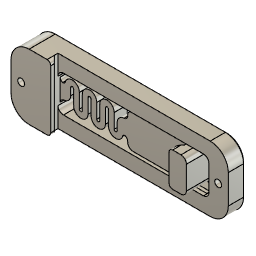
pcb_din_clip_x3 (Autodesk Fusion 360 design; units mm, degrees)
Autodesk Fusion 360 part; units mm, degrees
sketch "Sketch1" plane through (0, 0, 0) normal (0, 0, 1) x (1, 0, 0)
  line L0 (28.45, -9) -> (-28.45, -9)
  line L1 (-28.45, -9) -> (-28.45, 9)
  line L2 (-28.45, 9) -> (28.45, 9)
  line L3 (28.45, 9) -> (28.45, -9)
  line L4 (28.45, -9) -> (-28.45, 9) construction
  line L5 (-28.45, -9) -> (28.45, 9) construction
  dimension "d432" = 56.9
  dimension "d433" = 18
  constraint horizontal L0
  constraint perpendicular L0 L1
  constraint parallel L0 L2
  constraint parallel L1 L3
  constraint coincident L4 origin
  constraint coincident L5 origin
  measures "d432" distance of L1.end L2.end
  measures "d433" distance of L0.start L2.end
extrude "Extrude1" add sketch "Sketch1" along normal blind 7.6
sketch "Sketch2" plane through (0, 0, 7.6) normal (0, 0, 1) x (1, 0, 0)
  line L0 (28.45, 9) -> (-28.45, 9)
  line L1 (-28.45, 9) -> (-28.45, -9)
  line L2 (-28.45, -9) -> (28.45, -9)
  line L3 (28.45, -9) -> (28.45, 9)
  line L4 (-17.5, 9) -> (28.45, 9)
  line L5 (28.45, 9) -> (28.45, -9)
  line L6 (28.45, -9) -> (-17.5, -9)
  line L7 (-17.5, -9) -> (-17.5, 9)
  dimension "d436" = 10.95
  constraint horizontal L4
  constraint vertical L5
  constraint horizontal L6
  constraint vertical L7
  constraint coincident L2.end L3.start
  constraint coincident L0 L4.start
  measures "d436" distance of L1 L7
extrude "Extrude2" cut sketch "Sketch2" against normal blind 3 contours L0 L2 L3 L4 L5 L6 L7
sketch "Sketch3" plane through (0, -9, 0) normal (0, -1, 0) x (1, 0, 0)
  line L0 (28.45, 4.6) -> (-17.5, 4.6)
  line L1 (-17.5, 4.6) -> (-17.5, 7.6)
  line L2 (-17.5, 7.6) -> (-28.45, 7.6)
  line L3 (-28.45, 7.6) -> (-28.45, 0)
  line L4 (-28.45, 0) -> (28.45, 0)
  line L5 (28.45, 0) -> (28.45, 4.6)
  line L6 (-17.5, 6.6) -> (-18.5, 5.6)
  line L7 (-18.5, 5.6) -> (-18.5, 4.6)
  line L8 (-18.5, 4.6) -> (-17.5, 4.6)
  dimension "d439" = 1
  dimension "d440" = 1
  constraint coincident L1 L6.start
  constraint perpendicular L0 L7
  constraint coincident L0.end L1.start
  constraint perpendicular L1 L8
  constraint equal L7 L8
  measures "d439" distance of L7.end L0.end
  measures "d440" distance of L2 L6.start
extrude "Extrude3" cut sketch "Sketch3" against normal through all contours L1 L6 L7 L8
sketch "Sketch4" plane through (0, 0, 0) normal (0, 0, -1) x (-1, 0, 0)
  line L0 (28.45, 9) -> (-28.45, 9)
  line L1 (-28.45, 9) -> (-28.45, -9)
  line L2 (-28.45, -9) -> (28.45, -9)
  line L3 (28.45, -9) -> (28.45, 9)
  line L4 (-23.1, 5) -> (18.5, 5)
  line L5 (18.5, 5) -> (18.5, -5)
  line L6 (18.5, -5) -> (-23.1, -5)
  line L7 (-23.1, -5) -> (-23.1, 5)
  line L8 (-23.1, 5) -> (18.5, -5) construction
  line L9 (18.5, 5) -> (-23.1, -5) construction
  point P0 (-2.3, 0)
  dimension "d506" = 0.4
  constraint horizontal L4
  constraint perpendicular L4 L5
  constraint parallel L4 L6
  constraint parallel L5 L7
  constraint coincident L8 P0
  constraint coincident L9 P0
  constraint horizontal origin P0
  measures "d442" distance of L5.end L6.end
  measures "d443" distance of L1 L7
  measures "d453" distance of L4.start L6.end
extrude "Extrude4" cut sketch "Sketch4" against normal up to surface (4.6 mm away) contours L4 L5 L6 L7
ref_plane "WorkPlane1" through (21.5, 0, 3.8) normal (1, 0, 0) x (0, 1, 0)
sketch "Sketch5" plane through (21.5, 0, 2.1) normal (1, 0, 0) x (0, 0, -1)
  line L0 (0.4655, 6) -> (-0.4655, 6)
  line L1 (-0.4655, 6) -> (-0.4655, -6)
  line L2 (-0.4655, -6) -> (0.4655, -6)
  line L3 (0.4655, -6) -> (0.4655, 6)
  line L4 (0.4655, 6) -> (-0.4655, -6) construction
  line L5 (-0.4655, 6) -> (0.4655, -6) construction
  dimension "d447" = 0.931
  dimension "d448" = 12
  constraint horizontal L0
  constraint perpendicular L0 L1
  constraint parallel L0 L2
  constraint parallel L1 L3
  constraint coincident L4 origin
  constraint coincident L5 origin
  measures "d447" distance of L0.start L0.end
  measures "d448" distance of L0.start L2.end
extrude "Extrude5" cut sketch "Sketch5" against normal blind 15.5
chamfer "Chamfer1" distance 1 angle 45 4 edges at (13.75, 5, 2.5655) (13.75, 5, 1.6345) (13.75, -5, 2.5655) (13.75, -5, 1.6345)
sketch "Sketch6" plane through (0, 0, 0) normal (0, 0, -1) x (-1, 0, 0)
  line L0 (-23.1, -5) -> (-23.1, 5)
  line L1 (-23.1, 5) -> (18.5, 5)
  line L2 (18.5, 5) -> (18.5, -5)
  line L3 (18.5, -5) -> (-23.1, -5)
  line L4 (28.45, 9) -> (-28.45, 9)
  line L5 (-28.45, 9) -> (-28.45, -9)
  line L6 (-28.45, -9) -> (28.45, -9)
  line L7 (28.45, -9) -> (28.45, 9)
  line L8 (18.5, 5) -> (18.5, -5)
  line L9 (-23.1, 5) -> (18.5, 5)
  line L10 (18.5, -5) -> (-23.1, -5)
  line L11 (-23.1, -5) -> (-23.1, 5)
  line L12 (18.5, -2) -> (15.6, -2)
  line L13 (15.6, -2) -> (15.6, 2)
  line L14 (17.2, 2) -> (18.5, 2)
  line L15 (18.5, 2) -> (18.5, -2)
  line L16 (18.5, -2) -> (15.6, 2) construction
  line L17 (15.6, -2) -> (18.5, 2) construction
  line L18 (13.2, 2) -> (13.2, -2)
  line L19 (14.8, 2) -> (14.8, -2)
  arc A0 (10.8, -2) -> (14.8, -2) centre (12.8, -2) ccw
  arc A1 (17.2, 2) -> (13.2, 2) centre (15.2, 2) ccw
  line L20 (12.4, 2) -> (12.4, -2)
  line L21 (10.8, -2) -> (10.8, 2)
  arc A2 (12.4, -2) -> (13.2, -2) centre (12.8, -2) ccw
  arc A3 (12.4, 2) -> (8.4, 2) centre (10.4, 2) ccw
  line L22 (8.4, 2) -> (8.4, 2)
  arc A4 (15.6, 2) -> (14.8, 2) centre (15.2, 2) ccw
  arc A5 (10.8, 2) -> (10, 2) centre (10.4, 2) ccw
  line L23 (10, 2) -> (10, -2)
  line L24 (8.4, 2) -> (8.4, -2)
  arc A6 (6, -2) -> (10, -2) centre (8, -2) ccw
  line L25 (7.6, -2) -> (7.6, 2)
  line L26 (6, -2) -> (6, 2)
  arc A7 (7.6, -2) -> (8.4, -2) centre (8, -2) ccw
  line L27 (5.2, 2) -> (5.2, -2)
  line L28 (3.6, 2) -> (3.6, -2)
  line L29 (1.2, -2) -> (-0.1, -2)
  line L30 (-0.1, -2) -> (-0.1, 2)
  line L31 (-0.1, 2) -> (2.8, 2)
  line L32 (2.8, 2) -> (2.8, -2)
  line L33 (2.8, -2) -> (-0.1, 2) construction
  line L34 (-0.1, -2) -> (2.8, 2) construction
  arc A8 (1.2, -2) -> (5.2, -2) centre (3.2, -2) ccw
  arc A9 (7.6, 2) -> (3.6, 2) centre (5.6, 2) ccw
  arc A10 (6, 2) -> (5.2, 2) centre (5.6, 2) ccw
  arc A11 (2.8, -2) -> (3.6, -2) centre (3.2, -2) ccw
  arc A12 (10.8, 2.0006) -> (10, 1.9994) centre (10.4, 2) ccw
  arc A13 (10.8, 1.9994) -> (10.8, 2) centre (10.4, 2) ccw
  line L35 (-0.1, -4.7) -> (-19.9, -4.7)
  line L36 (-19.9, -4.7) -> (-19.9, 4.7)
  line L37 (-19.9, 4.7) -> (-0.1, 4.7)
  line L38 (-0.1, 4.7) -> (-0.1, -4.7)
  line L39 (-0.1, -4.7) -> (-19.9, 4.7) construction
  line L40 (-19.9, -4.7) -> (-0.1, 4.7) construction
  point P0 (17.05, 0)
  point P1 (1.35, 0)
  point P2 (-10, 0)
  dimension "d456" = 2.9
  dimension "d457" = 4
  dimension "d458" = 4
  dimension "d464" = 0.8
  dimension "d465" = 2.9
  dimension "d466" = 4
  dimension "d469" = 19.8
  dimension "d470" = 9.4
  constraint horizontal L12
  constraint perpendicular L12 L13
  constraint parallel L12 L14
  constraint parallel L13 L15
  constraint coincident L16 P0
  constraint coincident L17 P0
  constraint horizontal origin P0
  constraint coincident L8 L14.end
  constraint coincident L14 A1.centre
  constraint equal A0 A1
  constraint concentric A0 A2
  constraint coincident L12 A0.centre
  constraint tangent L18 A2
  constraint vertical L18
  constraint tangent L19 A0
  constraint vertical L19
  constraint concentric A3 A5
  constraint equal A1 A3
  constraint horizontal A1.centre A3.centre
  constraint tangent L20 A2
  constraint vertical L21
  constraint vertical L20
  constraint perpendicular L21 L22
  constraint horizontal A3.centre L21.end
  constraint horizontal L13.end L14.start
  constraint tangent L13 A4
  constraint horizontal L13.end A1.centre
  constraint tangent L19 A4
  constraint coincident A1.centre A4.centre
  constraint tangent L18 A1
  constraint coincident L21 A12.start
  constraint concentric A5 A12
  constraint concentric A6 A7
  constraint equal A0 A6
  constraint equal A2 A7
  constraint tangent L20 A3
  constraint tangent L21 A5
  constraint tangent A5 L23
  constraint vertical L24
  constraint horizontal A0.centre A6.centre
  constraint tangent L23 A6
  constraint vertical L23
  constraint concentric A9 A10
  constraint equal A3 A9
  constraint equal A5 A10
  constraint vertical L25
  constraint vertical L26
  constraint tangent A6 L26
  constraint tangent L25 A9
  constraint tangent L24 A7
  constraint tangent L25 A7
  constraint horizontal A3.centre A9.centre
  constraint vertical L27
  constraint vertical L28
  constraint tangent L27 A10
  constraint tangent L28 A9
  constraint horizontal L29
  constraint perpendicular L29 L30
  constraint parallel L29 L31
  constraint parallel L30 L32
  constraint coincident L33 P1
  constraint coincident L34 P1
  constraint horizontal origin P1
  constraint tangent L27 A8
  constraint equal A7 A11
  constraint coincident A8.centre A11.centre
  constraint tangent L28 A11
  constraint tangent L32 A11
  constraint horizontal L32.end L29.end
  constraint vertical L32.end L33.start
  constraint horizontal L29.start L32.end
  constraint coincident L23 A12.end
  constraint coincident L21 A13.start
  constraint concentric A12 A13
  constraint horizontal L35
  constraint perpendicular L35 L36
  constraint parallel L35 L37
  constraint parallel L36 L38
  constraint coincident L39 P2
  constraint coincident L40 P2
  constraint horizontal P1 P2
  constraint coincident L30.end L38
  measures "d456" distance of L12.start L12.end
  measures "d457" distance of L12.start L14.end
  measures "d458" diameter of A1
  measures "d464" diameter of A4
  measures "d465" distance of L32.end L29.end
  measures "d466" distance of L29.end L30.end
  measures "d469" distance of L36.end L37.end
  measures "d470" distance of L35.end L36.end
extrude "Extrude6" add sketch "Sketch6" against normal blind 4 contours L2 L8 L12 L13 L14 L15 L18 L19 A0 A1 L20 L21 A2 A3 A4 A5 L23 L24 A6 L25 L26 A7 L27 L28 L29 L30 L31 L32 A8 A9 A10 A11 A12 A13 L38 | L30 L35 L36 L37 L38
ref_plane "WorkPlane2" through (17.3, 0, 2) normal (1, 0, 0) x (0, 1, 0)
sketch "Sketch7" plane through (17.3, 0, 2) normal (1, 0, 0) x (0, 0, -1)
  line L0 (-0.4, -5.7) -> (0.2, -5.7)
  line L1 (0.2, -5.7) -> (0.2, 5.7)
  line L2 (0.2, 5.7) -> (-0.4, 5.7)
  line L3 (-0.4, 5.7) -> (-0.4, -5.7)
  line L4 (-0.4, -5.7) -> (0.2, 5.7) construction
  line L5 (0.2, -5.7) -> (-0.4, 5.7) construction
  line L6 (2, 4.7) -> (-2, 4.7)
  line L7 (2, -4.7) -> (-2, -4.7)
  line L8 (0.2, 5.7) -> (1.2, 4.7)
  line L9 (-0.4, 5.7) -> (-1.4, 4.7)
  line L10 (-1.4, 4.7) -> (-0.4, 4.7)
  line L11 (0.2, -5.7) -> (1.2, -4.7)
  line L12 (1.2, -4.7) -> (0.2, -4.7)
  line L13 (-0.4, -5.7) -> (-1.4, -4.7)
  line L14 (-1.4, -4.7) -> (-0.4, -4.7)
  point P0 (-0.1, 0)
  point P1 (-0.1, 0)
  dimension "d472" = 11.4
  dimension "d473" = 0.6
  dimension "d476" = 1
  dimension "d477" = 1
  dimension "d478" = 1
  dimension "d479" = 1
  constraint horizontal L0
  constraint perpendicular L0 L1
  constraint parallel L0 L2
  constraint parallel L1 L3
  constraint coincident L4 P1
  constraint coincident L5 P1
  constraint coincident P1 P0
  constraint coincident L6 L8.end
  constraint coincident L6 L9.end
  constraint coincident L3 L10.end
  constraint coincident L6 L10.end
  constraint coincident L7 L11.end
  constraint coincident L1 L12.end
  constraint coincident L7 L12.end
  constraint coincident L7 L13.end
  constraint coincident L3 L14.end
  constraint coincident L7 L14.end
  measures "d472" distance of L0.end L1.end
  measures "d473" distance of L0.start L0.end
  measures "d476" distance of L1 L8.end
  measures "d477" distance of L9.end L10.end
  measures "d478" distance of L11.end L12.end
  measures "d479" distance of L13.end L14.end
extrude "Extrude7" add sketch "Sketch7" against normal blind 9.3
sketch "Sketch8" plane through (0, 0, 4) normal (0, 0, 1) x (1, 0, 0)
  arc A0 (-5.2, -2) -> (-1.2, -2) centre (-3.2, -2) ccw
  line L0 (-1.2, -2) -> (0.1, -2)
  line L1 (0.1, -2) -> (0.1, -4.7)
  line L2 (0.1, -4.7) -> (19.9, -4.7)
  line L3 (19.9, -4.7) -> (19.9, 4.7)
  line L4 (19.9, 4.7) -> (0.1, 4.7)
  line L5 (0.1, 4.7) -> (0.1, 2)
  line L6 (0.1, 2) -> (-2.8, 2)
  line L7 (-2.8, 2) -> (-2.8, -2)
  arc A1 (-3.6, -2) -> (-2.8, -2) centre (-3.2, -2) ccw
  line L8 (-3.6, -2) -> (-3.6, 2)
  arc A2 (-3.6, 2) -> (-7.6, 2) centre (-5.6, 2) ccw
  line L9 (-7.6, 2) -> (-7.6, -2)
  arc A3 (-8.4, -2) -> (-7.6, -2) centre (-8, -2) ccw
  line L10 (-8.4, -2) -> (-8.4, 2)
  arc A4 (-8.4, 2) -> (-12.4, 2) centre (-10.4, 2) ccw
  line L11 (-12.4, 2) -> (-12.4, -2)
  arc A5 (-13.2, -2) -> (-12.4, -2) centre (-12.8, -2) ccw
  line L12 (-13.2, -2) -> (-13.2, 2)
  arc A6 (-13.2, 2) -> (-17.2, 2) centre (-15.2, 2) ccw
  line L13 (-17.2, 2) -> (-18.5, 2)
  line L14 (-18.5, 2) -> (-18.5, -2)
  line L15 (-18.5, -2) -> (-15.6, -2)
  line L16 (-15.6, -2) -> (-15.6, 2)
  arc A7 (-14.8, 2) -> (-15.6, 2) centre (-15.2, 2) ccw
  line L17 (-14.8, 2) -> (-14.8, -2)
  arc A8 (-14.8, -2) -> (-10.8, -2) centre (-12.8, -2) ccw
  line L18 (-10.8, -2) -> (-10.8, 1.9994)
  arc A9 (-10, 1.9994) -> (-10.8, 1.9994) centre (-10.4, 2) ccw
  line L19 (-10, 1.9994) -> (-10, -2)
  arc A10 (-10, -2) -> (-6, -2) centre (-8, -2) ccw
  line L20 (-6, -2) -> (-6, 2)
  arc A11 (-5.2, 2) -> (-6, 2) centre (-5.6, 2) ccw
  line L21 (-5.2, 2) -> (-5.2, -2)
  line L22 (19.9, 4.7) -> (15.1, 4.7)
  line L23 (15.1, 4.7) -> (15.1, -4.7)
  line L24 (15.1, -4.7) -> (19.9, -4.7)
  line L25 (19.9, -4.7) -> (19.9, 4.7)
  dimension "d480" = 4.8
  constraint horizontal L22
  constraint vertical L23
  constraint horizontal L24
  constraint vertical L25
  constraint coincident L3.end L4.start
  constraint coincident L2 L23.end
  measures "d480" distance of L3.end L22.end
extrude "Extrude8" add sketch "Sketch8" along normal blind 3.6 contours L2 L3 L4 L22 L23 L24 L25
sketch "Sketch9" plane through (0, -4.7, 0) normal (0, -1, 0) x (1, 0, 0)
  line L0 (8, 3.4) -> (17.3, 3.4)
  line L1 (17.3, 3.4) -> (17.3, 0.8)
  line L2 (17.3, 0.8) -> (8, 0.8)
  line L3 (8, 0.8) -> (8, 3.4)
  line L4 (0.1, 0) -> (19.9, 0)
  line L5 (19.9, 0) -> (19.9, 7.6)
  line L6 (19.9, 7.6) -> (15.1, 7.6)
  line L7 (15.1, 7.6) -> (15.1, 4)
  line L8 (15.1, 4) -> (0.1, 4)
  line L9 (0.1, 4) -> (0.1, 0)
  line L10 (15.1, 6.244) -> (16.5, 4.844)
  line L11 (16.5, 4.844) -> (16.5, 4)
  line L12 (16.5, 4) -> (15.1, 4)
  line L13 (15.1, 4) -> (15.1, 6.244)
  dimension "d483" = 0.844
  dimension "d484" = 1.4
  dimension "d485" = 45
  constraint coincident L7 L10.start
  constraint perpendicular L7 L12
  constraint perpendicular L8 L13
  constraint coincident L8 L7.end
  constraint vertical L11
  measures "d483" distance of L10.end L11.end
  measures "d484" distance of L11 L13
  measures "d485" angle of L10 L13
extrude "Extrude9" cut sketch "Sketch9" against normal up to surface (9.4 mm away) contours L7 L10 L11 L12 L13
hole "Hole2" at (-25.65, 0, 0) direction (0, 0, 1) diameter 1.9 end through all countersink diameter 2.7 countersink angle 90
hole "Hole1" at (25.65, 0, 0) direction (0, 0, 1) diameter 1.9 end through all countersink diameter 2.7 countersink angle 90
fillet "Fillet2" radius 1 12 edges at (-18.5, -2, 2) (-18.5, 2, 2) (0.1, -2, 2) (0.1, 2, 2) (15.1, 4.7, 6.922) (15.1, -4.7, 6.922) (-17.5, 9, 7.1) (-17.5, -9, 7.1) (21.5, -6, 2.1) (6, -6, 2.1) (6, 6, 2.1) (21.5, 6, 2.1)
fillet "Fillet2" radius 2 2 edges at (-15.6, -2, 2) (-2.8, 2, 2)
fillet "Fillet2" radius 0.5 2 edges at (-17.2, 2, 2) (-1.2, -2, 2)
fillet "Fillet2" radius 1.5 8 edges at (0.1, -4.7, 2) (0.1, 4.7, 2) (19.9, -4.7, 3.8) (19.9, 4.7, 3.8) (23.1, 5, 2.3) (23.1, -5, 2.3) (-18.5, -5, 2.3) (-18.5, 5, 2.3)
fillet "Fillet2" radius 5 4 edges at (-28.45, 9, 3.8) (-28.45, -9, 3.8) (28.45, 9, 2.3) (28.45, -9, 2.3)
chamfer "Chamfer2" distance 0.4 angle 45 58 edges at (-16.1624, -1.3921, 0) (-15.6, 0.9992, 0) (-15.2, 2.4, 0) (-14.8, 0, 0) (-12.8, -4, 0) (-10.8, -0.0003, 0) (-10.4, 2.4, 0) (-10, -0.0003, 0) (-8, -4, 0) (-6, 0, 0) (-5.6, 2.4, 0) (-5.2, 0, 0) (-3.4098, -3.989, 0) (-1.0092, -2.0909, 0) (-0.0969, -2.4042, 0) (0.1, -3.1, 0) (0.5393, -4.2607, 0) (10, -4.7, 0) (19.4606, -4.2607, 0) (19.9, 0, 0) (19.4606, 4.2607, 0) (10, 4.7, 0) (0.5393, 4.2607, 0) (0.1, 3.1, 0) (-0.1812, 2.3048, 0) (-2.2376, 1.3921, 0) (-2.8, -0.9992, 0) (-3.2, -2.4, 0) (-3.6, 0, 0) (-5.6, 4, 0) (-7.6, 0, 0) (-8, -2.4, 0) (-8.4, 0, 0) (-10.4, 4, 0) (-12.4, 0, 0) (-12.8, -2.4, 0) (-13.2, 0, 0) (-14.9902, 3.989, 0) (-17.3909, 2.0909, 0) (-18.3031, 2.4042, 0) (-18.5, 3.25, 0) (-18.0607, 4.5607, 0) (2.3, 5, 0) (22.6607, 4.5607, 0) (23.1, 0, 0) (22.6607, -4.5607, 0) (2.3, -5, 0) (-18.0607, -4.5607, 0) (-18.5, -3.25, 0) (-18.2188, -2.3048, 0) (-26.9855, -7.5355, 0) (0, -9, 0) (26.9855, -7.5355, 0) (28.45, 0, 0) (26.9855, 7.5355, 0) (0, 9, 0) (-26.9855, 7.5355, 0) (-28.45, 0, 0)
equation "d440 = d439"
equation "d477 = d476"
equation "d478 = d476"
equation "d479 = d476"
equation "d485 = 45 °"
